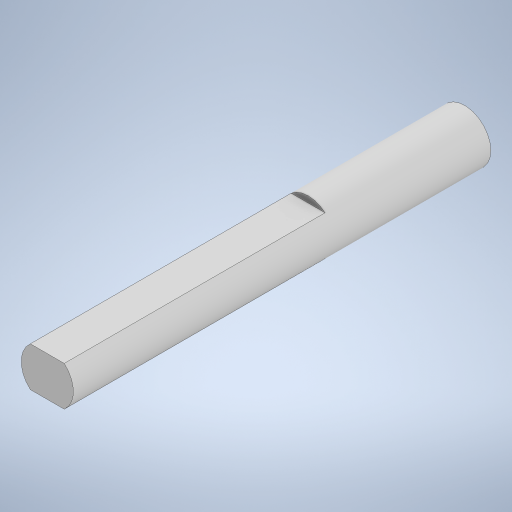
# Autodesk Inventor part: ShaftRoda
Saved by Autodesk Inventor 2024 (Build 280153000, 153)
## iProperties
Created: 2025-12-11
Part Number: ShaftRoda
Material: Generic
Document SubType Name: Modeling
Designer: risda
Density: 1 g/cm^3
Appearance: Default
Author: risda
Autodesk Inventor part; units mm, degrees
ref_plane "YZ Plane" through (0, 0, 0) normal (1, 0, 0) x (0, 1, 0)
ref_plane "XZ Plane" through (0, 0, 0) normal (0, 1, 0) x (-1, 0, 0)
ref_plane "XY Plane" through (0, 0, 0) normal (0, 0, 1) x (1, 0, 0)
sketch "Sketch1" plane through (0, 0, 0) normal (0, 0, 1) x (1, 0, 0)
  circle A0 centre (0, 0) radius 2.5
  dimension "d0" = 5
  constraints: 1 centre point, 1 coincident
  measures "d0" diameter of A0
extrude "Extrusion1" add sketch "Sketch1" along normal blind 10 and the other way blind 5
sketch "Sketch2" plane through (0, 0, 10) normal (0, 0, 1) x (1, 0, 0)
  line L0 (0, 0) -> (0, 1.9)
  circle A0 centre (0, 0) radius 2.5 projected
  line L1 (0, 0) -> (0, -1.9)
  line L2 (0, -1.9) -> (1.6248, -1.9)
  line L3 (0, -1.9) -> (-1.6248, -1.9)
  line L4 (0, 1.9) -> (1.6248, 1.9)
  line L5 (0, 1.9) -> (-1.6248, 1.9)
  circle A1 centre (0, 0) radius 2.5
  dimension "d3" = 1.9
  dimension "d4" = 1.9
  constraints: 12 end point, 4 point on circle, 2 horizontal, 2 vertical, 1 centre point, 1 coincident, 1 concentric, 1 perpendicular, 1 point on line
  measures "d3" distance of L0.start L0.end
  measures "d4" distance of L1.start L1.end
extrude "Extrusion2" add sketch "Sketch2" along normal blind 25 contours L1 L3 A0 L5 L0 | L0 L4 A0 L2 L1
body "Solid1"
